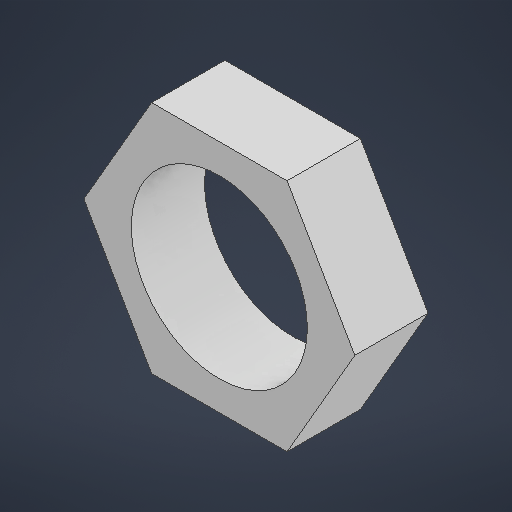
# Autodesk Inventor part: Bolt
Saved by Autodesk Inventor 2026 (Build 300175000, 175)
## iProperties
Created: 2025-05-08
Part Number: Bolt
Material: Generic
Document SubType Name: Modeling
Designer: Ritul Kumari
Density: 1 g/cm^3
Appearance: Default
Author: Ritul Kumari
Autodesk Inventor part; units mm, degrees
ref_plane "YZ Plane" through (0, 0, 0) normal (1, 0, 0) x (0, 1, 0)
ref_plane "XZ Plane" through (0, 0, 0) normal (0, 1, 0) x (-1, 0, 0)
ref_plane "XY Plane" through (0, 0, 0) normal (0, 0, 1) x (1, 0, 0)
sketch "Sketch1" plane through (0, 0, 0) normal (0, 0, 1) x (1, 0, 0)
  line L0 (234.6351, 0) -> (117.3176, -203.2)
  line L1 (117.3176, -203.2) -> (-117.3176, -203.2)
  line L2 (-117.3176, -203.2) -> (-234.6351, 0)
  line L3 (-234.6351, 0) -> (-117.3176, 203.2)
  line L4 (-117.3176, 203.2) -> (117.3176, 203.2)
  line L5 (117.3176, 203.2) -> (234.6351, 0)
  circle A0 centre (0, 0) radius 152.4
  point P0 (0, -203.2)
  point P1 (0, 203.2)
  dimension "d0" = 406.4
  dimension "d1" = 304.8
  constraints: 12 end point, 2 coincident, 2 midpoint, 1 centre point, 13 other
  measures "d0" distance of point (0, -203.2) point (0, 203.2)
  measures "d1" diameter of A0
extrude "Extrusion1" add sketch "Sketch1" along normal blind 127
body "Solid1"
